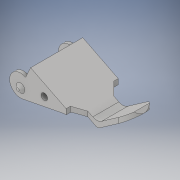
# Autodesk Inventor part: PKWS1-HOOK
Saved by Autodesk Inventor 2019 (Build 230136000, 136)
## iProperties
Created: 2024-01-04
Part Number: PKWS1-HOOK
Material: Generic
Catalog Web Link: www.cadenas.de
Description: PKWS-HOOK-Snap Locks
Vendor: MISUMI
Document SubType Name: Modeling
Designer: psAdmin
Manufacturer: MISUMI
Mass: 0.46127 g
Surface Area: 7.80873 cm^2
Volume: 0.46127 cm^3
Density: 1 g/cm^3
Appearance: PSOLRGB-175-175-175
Category: PARTsolutions
Company: MISUMI
Title: PKWS1-HOOK
Author: Cadenas PARTsolutions
Comments: Snap Locks
PSOL_IDENT_0: {$CADENAS_DATA/23d-libs/misumi/metric/44_handles_hinges/pkws_hook.prj},163 {VTYP=3D},{NB=PKWS1-HOOK}
PSOL_IDENT_1: ,{LINA=PKWS1-HOOK},{NN=PKWS-HOOK},{DATE=04.06.2021 03:58:35},{GEOMDATE=17.02.2014 00:00:00},{VERSION=
PSOL_IDENT_2: },{LINEID=10},{WBVAR=},{WBNUMERIC=}  {NB=PKWS1-HOOK},{LINA=PKWS1-HOOK},{KT=DUMMY},{PN=PKWS1},{NO=1},
PSOL_IDENT_3: {TL=49 (5)},{MASS=11},{PPATH=assemblies_pkws\\pkws_templ.prj},{ANGLE=10.015}
NB: PKWS1-HOOK
NN: PKWS-HOOK
NT: Snap Locks
NBSYN: $PN.-HOOK
LINA: PKWS1-HOOK
CATALOG: Misumi
PN: PKWS1
NO: 1
TL: 49 (5)
MASS: 11
ANGLE: 10.015
SUPPLIER: MISUMI
ARTICLENO: PKWS1-HOOK
BOMINFO: PKWS1-HOOK
CREATOR: CADENAS GmbH
Autodesk Inventor part; units mm, degrees
sketch "Sketch_1" plane through (0, 0, 0) normal (0, 0, 1) x (1, 0, 0)
  arc A0 (3.6737, 5.7073) -> (2.9784, 1.0462) centre (2.5, 3.5) ccw
  line L0 (2.9784, 1.0462) -> (12.3318, 2.8697)
  arc A1 (13.6089, 2.6955) -> (12.3318, 2.8697) centre (12.7145, 0.9067) ccw
  line L1 (13.6089, 2.6955) -> (16.8654, 1.0673)
  arc A2 (16.8654, 1.0673) -> (17.6821, 1.1275) centre (17.2232, 1.7828) ccw
  line L2 (17.6821, 1.1275) -> (25, 6.2516)
  line L3 (25, 6.2516) -> (24.4264, 7.0707)
  line L4 (24.4264, 7.0707) -> (18.182, 2.6984)
  arc A3 (16.1405, 2.5478) -> (18.182, 2.6984) centre (17.0349, 4.3367) ccw
  line L5 (16.1405, 2.5478) -> (4.8361, 8.2)
  line L6 (4.8361, 8.2) -> (3.6737, 5.7073)
  circle A4 centre (8, 4) radius 0.75
  constraints: 14 end point, 8 point on circle, 5 centre point
extrude "Extrusion1" add sketch "Sketch_1" along normal mid plane 12
sketch "Sketch_2" plane through (0, 0, 0) normal (0, 0, 1) x (1, 0, 0)
  circle A0 centre (2.5, 3.5) radius 3.8829
  constraints: 1 centre point
extrude "Extrusion2" cut sketch "Sketch_2" along normal mid plane 10.5
sketch "Sketch_3" plane through (0, 0, 0) normal (0, 1, 0) x (-1, 0, 0)
  line L0 (-13, -5) -> (-15, -3)
  line L1 (-15, -3) -> (-22, -3)
  arc A0 (-22, 3) -> (-22, -3) centre (-22, 0) ccw
  line L2 (-22, 3) -> (-15, 3)
  line L3 (-15, 3) -> (-13, 5)
  line L4 (-13, 5) -> (-13, 6)
  line L5 (-13, 6) -> (-30, 6)
  line L6 (-30, 6) -> (-30, -6)
  line L7 (-30, -6) -> (-13, -6)
  line L8 (-13, -6) -> (-13, -5)
  constraints: 18 end point, 2 point on circle, 1 centre point
extrude "Extrusion3" cut sketch "Sketch_3" along normal blind 15
sketch "Sketch_4" plane through (2.5, 0, 0) normal (1, 0, 0) x (0, 0, -1)
  line L0 (6.75, 3) -> (-6.75, 3)
  arc A0 (-6.6154, 3.3413) -> (-6.75, 3) centre (-6.25, 3) ccw
  line L1 (-6.6154, 3.3413) -> (-6, 4)
  line L2 (-6, 4) -> (6, 4)
  line L3 (6, 4) -> (6.6154, 3.3413)
  arc A1 (6.75, 3) -> (6.6154, 3.3413) centre (6.25, 3) ccw
  line L4 (6.75, 3) -> (-6.75, 3)
  constraints: 10 end point, 4 point on circle, 2 centre point
revolve "Revolution1" add sketch "Sketch_4" angle 360 about axis through (2.5, 3, -6.75) along (0, 0, -1)
ref_plane "A_XY" through (2.5, 3, 0) normal (0, 0, 1) x (1, 0, 0)
ref_plane "A_YZ" through (2.5, 3, 0) normal (1, 0, 0) x (0, 1, 0)
ref_plane "A_ZX" through (2.5, 3, 0) normal (0, 1, 0) x (0, 0, 1)
ref_plane "B_XY" through (8, 4, 0) normal (0, 0, 1) x (1, 0, 0)
ref_plane "B_YZ" through (8, 4, 0) normal (1, 0, 0) x (0, 1, 0)
ref_plane "B_ZX" through (8, 4, 0) normal (0, 1, 0) x (0, 0, 1)
body "Solid1"
